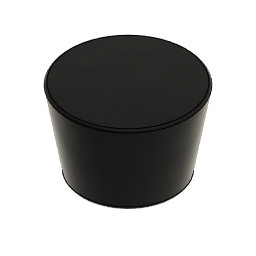
3030 Leveling Feet Assembly (Autodesk Fusion 360 archive; units mm, degrees)
design "Rubber Foot"
Autodesk Fusion 360 part; units mm, degrees
sketch "Skizze1" plane through (0, 0, 0) normal (0, 1, 0) x (1, 0, 0)
  line L0 (0, 0) -> (12, 0)
  line L1 (12, 0) -> (9.1788, 16)
  line L2 (9.1788, 16) -> (4, 16)
  line L3 (4, 16) -> (4, 10)
  line L4 (4, 10) -> (0, 10)
  line L5 (0, 10) -> (0, 0)
  dimension "d1" = 12
  dimension "d2" = 80
  dimension "d3" = 16
  dimension "d4" = 4
  dimension "d5" = 6
  constraint coincident L0.start L5.end
  constraint horizontal L0
  constraint parallel L0 L2
  constraint perpendicular L2 L3
  constraint perpendicular L3 L4
  constraint perpendicular L4 L5
  measures "d1" distance of L0.start L0.end
  measures "d2" angle of L0 L1
  measures "d3" distance of L0 L2
  measures "d4" distance of L3.end L4.end
  measures "d5" distance of L2.end L3.end
revolve "Drehen1" add sketch "Skizze1" angle 360 about axis through (0, 0, 1.75) along (0, 0, 1)
fillet "Abrundung1" radius 0.4 1 edges at (-11.1879, -4.3394, 0)
fillet "Abrundung2" radius 1 2 edges at (-3.7293, -1.4465, -16) (-8.5576, -3.3192, -16)

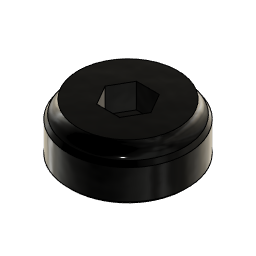
design "Leveling Foot Base"
Autodesk Fusion 360 part; units mm, degrees
sketch "sketch 611" plane through (0, 0, -25.25) normal (0, 0, -1) x (1, 0, 0)
  line L0 (-17.8637, 12.9787) -> (-22.0807, 0)
  line L1 (-22.0807, 0) -> (-17.8637, -12.9787)
  line L2 (-17.8637, -12.9787) -> (-6.8233, -21)
  line L3 (-6.8233, -21) -> (6.8233, -21)
  line L4 (6.8233, -21) -> (17.8637, -12.9787)
  line L5 (17.8637, -12.9787) -> (22.0807, 0)
  line L6 (22.0807, 0) -> (17.8637, 12.9787)
  line L7 (17.8637, 12.9787) -> (6.8233, 21)
  line L8 (6.8233, 21) -> (-6.8233, 21)
  line L9 (-6.8233, 21) -> (-17.8637, 12.9787)
extrude "Extrude1" add sketch "sketch 611" along normal blind 5 and the other way blind 5
sketch "sketch 651" plane through (0, 0, -20.25) normal (0, 0, 1) x (-1, 0, 0)
  line L0 (-2.3094, 4) -> (-4.6188, 0)
  line L1 (-4.6188, 0) -> (-2.3094, -4)
  line L2 (-2.3094, -4) -> (2.3094, -4)
  line L3 (2.3094, -4) -> (4.6188, 0)
  line L4 (4.6188, 0) -> (2.3094, 4)
  line L5 (2.3094, 4) -> (-2.3094, 4)
extrude "Extrude3" cut sketch "sketch 651" against normal blind 5
sketch "sketch 678" plane through (0, 0, -20.25) normal (0, 0, 1) x (-1, 0, 0)
  circle A0 centre (0, 0) radius 10
  line L0 (17.8637, -12.9787) -> (22.0807, 0)
  line L1 (22.0807, 0) -> (17.8637, 12.9787)
  line L2 (17.8637, 12.9787) -> (6.8233, 21)
  line L3 (6.8233, 21) -> (-6.8233, 21)
  line L4 (-6.8233, 21) -> (-17.8637, 12.9787)
  line L5 (-17.8637, 12.9787) -> (-22.0807, 0)
  line L6 (-22.0807, 0) -> (-17.8637, -12.9787)
  line L7 (-17.8637, -12.9787) -> (-6.8233, -21)
  line L8 (-6.8233, -21) -> (6.8233, -21)
  line L9 (6.8233, -21) -> (17.8637, -12.9787)
extrude "Extrude4" cut sketch "sketch 678" against normal blind 3
fillet "Fillet1" radius 3 1 edges at (-9.3233, -3.6162, -23.25)
fillet "Fillet2" radius 1 10 edges at (22.0807, 0, -26.75) (17.8637, -12.9787, -26.75) (6.8233, -21, -26.75) (-6.8233, -21, -26.75) (-17.8637, -12.9787, -26.75) (17.8637, 12.9787, -26.75) (-22.0807, 0, -26.75) (-17.8637, 12.9787, -26.75) (-6.8233, 21, -26.75) (6.8233, 21, -26.75)
sketch "sketch 720" plane through (0, 0, -30.25) normal (0, 0, -1) x (1, 0, 0)
  circle A0 centre (0, 0) radius 17.5
extrude "Extrude5" add sketch "sketch 720" along normal blind 1
extrude "Extrude6" cut 1 faces at (4.4225, 5.9212, -31.25) along direction (0, 0, 1) blind 1
sketch "Sketch1" plane through (0, 0, -30.25) normal (0, 0, -1) x (1, 0, 0)
  arc A0 (6.4984, -21) -> (7.0862, -20.809) centre (6.4984, -20) ccw
  line L0 (7.0862, -20.809) -> (17.6008, -13.1697)
  arc A1 (17.6008, -13.1697) -> (17.9641, -12.6697) centre (17.013, -12.3607) ccw
  line L1 (17.9641, -12.6697) -> (21.9803, -0.309)
  arc A2 (21.9803, -0.309) -> (21.9803, 0.309) centre (21.0292, 0) ccw
  line L2 (21.9803, 0.309) -> (17.9641, 12.6697)
  arc A3 (17.9641, 12.6697) -> (17.6008, 13.1697) centre (17.013, 12.3607) ccw
  line L3 (17.6008, 13.1697) -> (7.0862, 20.809)
  arc A4 (7.0862, 20.809) -> (6.4984, 21) centre (6.4984, 20) ccw
  line L4 (6.4984, 21) -> (-6.4984, 21)
  arc A5 (-6.4984, 21) -> (-7.0862, 20.809) centre (-6.4984, 20) ccw
  line L5 (-7.0862, 20.809) -> (-17.6008, 13.1697)
  arc A6 (-17.6008, 13.1697) -> (-17.9641, 12.6697) centre (-17.013, 12.3607) ccw
  line L6 (-17.9641, 12.6697) -> (-21.9803, 0.309)
  arc A7 (-21.9803, 0.309) -> (-21.9803, -0.309) centre (-21.0292, 0) ccw
  line L7 (-21.9803, -0.309) -> (-17.9641, -12.6697)
  arc A8 (-17.9641, -12.6697) -> (-17.6008, -13.1697) centre (-17.013, -12.3607) ccw
  line L8 (-17.6008, -13.1697) -> (-7.0862, -20.809)
  arc A9 (-7.0862, -20.809) -> (-6.4984, -21) centre (-6.4984, -20) ccw
  line L9 (-6.4984, -21) -> (6.4984, -21)
  circle A10 centre (0, 0) radius 12
  dimension "d1" = 24
  constraint coincident A10.centre origin
  measures "d1" diameter of A10
extrude "Extrude7" cut sketch "Sketch1" against normal blind 10
chamfer "Chamfer1" distance 0.6 angle 45 2 edges at (-11.1879, -4.3394, -23.0784) (-11.1879, 4.3394, -30.25)
